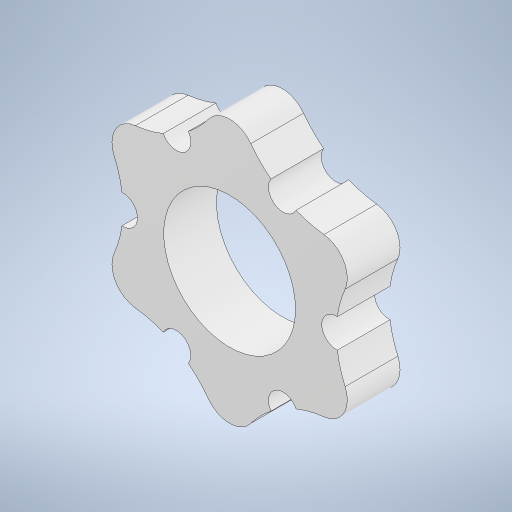
# Autodesk Inventor part: Gyro Core
Saved by Autodesk Inventor 2023.2 (Build 272271000, 271)
## iProperties
Created: 2023-06-11
Part Number: Gyro Core
Material: UHMW, White
Document SubType Name: Modeling
Designer: Nathan Cai
Density: 0.94 g/cm^3
Appearance: Smooth - White
Mass: 2.41132 g
Surface Area: 18.3446 cm^2
Volume: 2.56524 cm^3
Author: Nathan Cai
Autodesk Inventor part; units mm, degrees
ref_plane "YZ Plane" through (0, 0, 0) normal (1, 0, 0) x (0, 1, 0)
ref_plane "XZ Plane" through (0, 0, 0) normal (0, 1, 0) x (-1, 0, 0)
ref_plane "XY Plane" through (0, 0, 0) normal (0, 0, 1) x (1, 0, 0)
sketch "Sketch1" plane through (0, 0, 0) normal (0, 0, 1) x (1, 0, 0)
  circle A0 centre (0, 0) radius 7.9375
  circle A1 centre (0, 0) radius 15.875 construction
  line L0 (0, 0) -> (0, 15.875) construction
  circle A2 centre (0, 12.7) radius 3.175
  circle A3 centre (-10.9985, 6.35) radius 3.175
  circle A4 centre (-10.9985, -6.35) radius 3.175
  circle A5 centre (0, -12.7) radius 3.175
  circle A6 centre (10.9985, -6.35) radius 3.175
  circle A7 centre (10.9985, 6.35) radius 3.175
  arc A8 (-11.3536, 9.5051) -> (-2.5548, 14.5851) centre (-12.7741, 22.1254) ccw
  circle A9 centre (-6.4241, 11.1269) radius 1.7526
  circle A10 centre (-12.8482, 0) radius 1.7526
  arc A11 (-13.9085, -5.08) -> (-13.9085, 5.08) centre (-25.5482, 0) ccw
  circle A12 centre (-6.4241, -11.1269) radius 1.7526
  arc A13 (-2.5548, -14.5851) -> (-11.3536, -9.5051) centre (-12.7741, -22.1254) ccw
  circle A14 centre (6.4241, -11.1269) radius 1.7526
  arc A15 (11.3536, -9.5051) -> (2.5548, -14.5851) centre (12.7741, -22.1254) ccw
  circle A16 centre (12.8482, 0) radius 1.7526
  arc A17 (13.9085, 5.08) -> (13.9085, -5.08) centre (25.5482, 0) ccw
  circle A18 centre (6.4241, 11.1269) radius 1.7526
  arc A19 (2.5548, 14.5851) -> (11.3536, 9.5051) centre (12.7741, 22.1254) ccw
  point P0 (-13.9085, 5.08)
  point P1 (-12.9691, 1.7484)
  point P2 (-12.9691, -1.7484)
  point P3 (-13.9085, -5.08)
  point P4 (-11.3536, -9.5051)
  point P5 (-7.9987, -10.3574)
  point P6 (-4.9704, -12.1058)
  point P7 (-2.5548, -14.5851)
  point P8 (2.5548, -14.5851)
  point P9 (4.9704, -12.1058)
  point P10 (7.9987, -10.3574)
  point P11 (11.3536, -9.5051)
  point P12 (13.9085, -5.08)
  point P13 (12.9691, -1.7484)
  point P14 (12.9691, 1.7484)
  point P15 (13.9085, 5.08)
  point P16 (11.3536, 9.5051)
  point P17 (7.9987, 10.3574)
  point P18 (4.9704, 12.1058)
  point P19 (2.5548, 14.5851)
  point P20 (-4.9704, 12.1058)
  point P21 (-7.9987, 10.3574)
  dimension "d1" = 31.75
  dimension "d2" = 6.35
  dimension "d0" = 15.875
  dimension "d5" = 360
  dimension "d7" = 12.7
  dimension "d8" = 3.5052
  dimension "d11" = 360
  constraints: 17 centre point, 13 point on circle, 2 coincident, 2 end point, 1 point on line, 1 vertical, 1 vertical alignment, 60 other
  measures "d0" diameter of A0
  measures "d7" radius of A8
  measures "d8" diameter of A9
extrude "Extrusion1" add sketch "Sketch1" along normal blind 6.35 contours A2 | A2 A19 A18 A7 A17 A16 A6 A15 A14 A5 A13 A12 A4 A11 A10 A3 A8 A9 | A7 | A3 | A6 | A4 | A5
equation "\"d1\" = Brass_ID"
equation "\"Brass_ID\" = 31.75"
body "Solid1"
